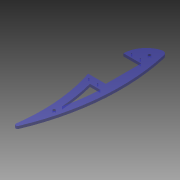
# Autodesk Inventor part: Tibia
Saved by Autodesk Inventor 2015 SP2 (Build 190223200, 223)
## iProperties
Created: 2015-10-11
Part Number: Tibia
Material: Generic
Document SubType Name: Modeling
Designer: styku
Density: 1 g/cm^3
Appearance: Blue
Mass: 5.37381 g
Surface Area: 53.342 cm^2
Volume: 5.37381 cm^3
Author: styku
Autodesk Inventor part; units mm, degrees
ref_plane "YZ Plane" through (0, 0, 0) normal (1, 0, 0) x (0, 1, 0)
ref_plane "XZ Plane" through (0, 0, 0) normal (0, 1, 0) x (-1, 0, 0)
ref_plane "XY Plane" through (0, 0, 0) normal (0, 0, 1) x (1, 0, 0)
sketch "Sketch1" plane through (0, 0, 0) normal (0, 0, 1) x (1, 0, 0)
  line L0 (0, 102) -> (0, -107) construction
  line L1 (119, 0) -> (-122, 0) construction
  line L2 (-10, 20) -> (10, 20)
  line L3 (10, 20) -> (10, -20)
  line L4 (10, -20) -> (-10, -20)
  arc A0 (8.5715, 44.7916) -> (-10, 20) centre (15.9997, 19.8753) ccw
  arc A1 (1.8457, -110.7703) -> (14.8748, 41.1118) centre (-228.8662, -14.4789) ccw
  arc A2 (14.8748, 41.1118) -> (8.5715, 44.7916) centre (10, 40) ccw
  circle A3 centre (5, 24.25) radius 0.5
  circle A4 centre (-5, 24.25) radius 0.5
  arc A5 (-1.981, -109.7248) -> (-10, -20) centre (-200.0791, -82.2088) ccw
  arc A6 (-1.981, -109.7248) -> (1.8457, -110.7703) centre (0, -110) ccw
  arc A7 (7.3645, -67.0056) -> (12.6978, -29) centre (-228.8662, -14.4789) ccw
  arc A8 (7.3645, -67.0056) -> (1, -29) centre (-200.0791, -82.2088) ccw
  line L5 (12.6978, -29) -> (1, -29)
  circle A9 centre (5, -24.25) radius 0.5
  circle A10 centre (-5, -24.25) radius 0.5
  circle A11 centre (6.5, -75.0056) radius 1.5
  circle A12 centre (6.5, 33) radius 1.5
  point P0 (0, 0)
  dimension "d0" = 20
  dimension "d1" = 40
  dimension "d2" = 5
  dimension "d3" = 26
  dimension "d4" = 10
  dimension "d5" = 1
  dimension "d6" = 4.25
  dimension "d7" = 5
  dimension "d8" = 20
  dimension "d9" = 250
  dimension "d10" = 10
  dimension "d11" = 20
  dimension "d12" = 2
  dimension "d13" = 150
  dimension "d14" = 200
  dimension "d15" = 208
  dimension "d16" = 242
  dimension "d17" = 9
  dimension "d20" = 3
  dimension "d21" = 8
  dimension "d22" = 6.5
  dimension "d23" = 3
  dimension "d24" = 6.5
  dimension "d25" = 13
  constraints: 14 point on circle, 13 centre point, 12 end point, 4 tangent, 3 horizontal, 3 symmetric about line, 3 vertical, 2 concentric, 2 parallel, 1 perpendicular, 1 point on line, 3 other
  measures "d0" distance of L2.start L2.end
  measures "d1" distance of L2.end L3.end
  measures "d2" radius of A2
  measures "d3" radius of A0
  measures "d4" distance between parallel lines of L0 L3
  measures "d5" diameter of A3
  measures "d6" distance from line of L2 A3.centre
  measures "d7" distance from line of L3 A3.centre
  measures "d8" distance between parallel lines of L1 L2
  measures "d9" radius of A1
  measures "d10" distance from line of L0 A2.centre
  measures "d11" distance from line of L2 A2.centre
  measures "d12" radius of A6
  measures "d13" vertical distance of A2.centre A6.centre
  measures "d14" radius of A5
  measures "d15" radius of A8
  measures "d16" radius of A7
  measures "d17" distance between parallel lines of L4 L5
  measures "d20" diameter of A11
  measures "d21" vertical distance of A7.start A11.centre
  measures "d22" distance from line of A11.centre L0
  measures "d23" diameter of A12
  measures "d24" distance from line of L0 A12.centre
  measures "d25" distance from line of L2 A12.centre
extrude "Extrusion2" add sketch "Sketch1" along normal blind 3
body "Solid2"
